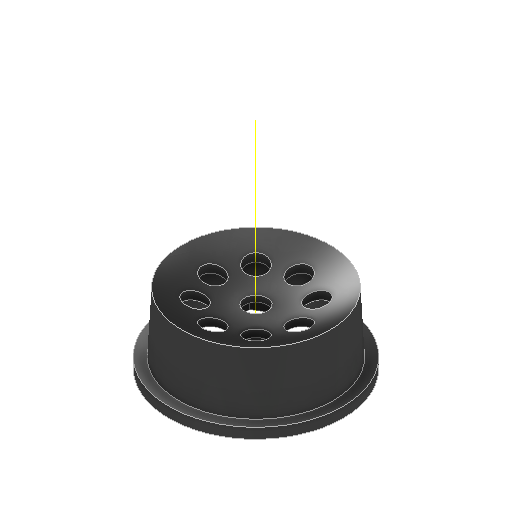
# Autodesk Inventor part: RIM ver 1
Saved by Autodesk Inventor 2023 (Build 270158000, 158)
## iProperties
Created: 2023-03-21
Part Number: RIM ver 1
Material: Generic
Document SubType Name: Modeling
Designer: Juyoung Han
Density: 1 g/cm^3
Appearance: Glossy - Black
Author: Juyoung Han
Autodesk Inventor part; units mm, degrees
ref_plane "YZ Plane" through (0, 0, 0) normal (1, 0, 0) x (0, 1, 0)
ref_plane "XZ Plane" through (0, 0, 0) normal (0, 1, 0) x (-1, 0, 0)
ref_plane "XY Plane" through (0, 0, 0) normal (0, 0, 1) x (1, 0, 0)
sketch "Sketch1" plane through (0, 0, 0) normal (0, 0, 1) x (1, 0, 0)
  line L0 (68.5, -28.5) -> (70.5, -28.5)
  line L1 (70.5, -28.5) -> (70.5, -20)
  line L2 (68.5, -28.5) -> (68.5, -22.5)
  line L3 (68.5, -22.5) -> (66.5, -22.5)
  line L4 (66.5, -22.5) -> (66.5, -24.5)
  line L5 (66.5, -24.5) -> (59.5, -24.5)
  line L6 (70.5, -20) -> (62.5, -20)
  line L7 (62.5, -20) -> (59.9389, 28.8689)
  line L8 (62.5, -20) -> (70.5, -20) construction
  line L9 (9.25, 16.5) -> (9.25, 11.5)
  line L10 (19, 11.5) -> (19, 3.5)
  line L11 (12, 3.5) -> (12, 11.5)
  arc A0 (9.25, 16.5) -> (59.9582, 28.5) centre (9.25, 129.6385) ccw
  line L12 (12, 11.5) -> (9.25, 11.5)
  line L13 (9.25, 11.5) -> (12, 11.5)
  line L14 (19, 3.5) -> (12, 3.5)
  line L15 (59.5, -24.5) -> (57.5607, 12.5037)
  line L16 (59.5, -24.5) -> (96.5545, -24.5) construction
  line L17 (57.5607, 12.5037) -> (57.1249, 20.8194)
  arc A1 (19, 11.5) -> (57.1249, 20.8194) centre (19, 94.1424) ccw
  line L18 (0, -60.1277) -> (0, 161.2662) projected
  point P0 (0, 0)
  point P1 (9.25, 14)
  dimension "d4" = 6
  dimension "d5" = 2
  dimension "d6" = 2
  dimension "d7" = 7
  dimension "d8" = 8
  dimension "d9" = 8.5
  dimension "d10" = 2
  dimension "d11" = 48.936
  dimension "d12" = 93
  dimension "d17" = 8
  dimension "d23" = 93
  constraints: 36 end point, 5 perpendicular, 4 horizontal, 4 point on circle, 2 centre point, 2 point on line, 1 equal length, 1 midpoint, 1 parallel, 1 vertical
  measures "d4" distance of L0.start L2.end
  measures "d5" distance of L2.end L3.end
  measures "d6" distance of L3.end L4.end
  measures "d7" distance of L4.end L5.end
  measures "d8" distance of L1.end L6.end
  measures "d9" distance between parallel lines of L0 L6
  measures "d10" distance between parallel lines of L1 L2
  measures "d11" distance of L6.end L7.end
  measures "d12" angle of L8 L7
  measures "d17" distance of L10.start L10.end
  measures "d23" angle of L16 L15
revolve "Revolution1" add sketch "Sketch1" angle 360 about axis through (0, -10, 0) along (0, 1, 0)
sketch "Sketch2" plane through (0, 3.5, 0) normal (0, -1, 0) x (1, 0, 0)
  circle A0 centre (0, 0) radius 12 projected
  circle A1 centre (0, 0) radius 19 projected
  line L0 (12, 6.9282) -> (12, -6.9282)
  line L1 (12, -6.9282) -> (0, -13.8564)
  line L2 (0, -13.8564) -> (-12, -6.9282)
  line L3 (-12, -6.9282) -> (-12, 6.9282)
  line L4 (-12, 6.9282) -> (0, 13.8564)
  line L5 (0, 13.8564) -> (12, 6.9282)
  point P0 (10.3923, -6)
  dimension "d47" = 24
  dimension "d48" = 0
  constraints: 12 end point, 2 coincident, 15 other
  measures "d47" distance between parallel lines of L4 L1
  measures "d48" horizontal distance of point (0, 0) L4.end
sketch "Sketch3" plane through (0, 3.5, 0) normal (0, -1, 0) x (1, 0, 0)
  circle A0 centre (0, 35) radius 8.75
  circle A1 centre (-24.7487, 24.7487) radius 8.75
  circle A2 centre (-35, 0) radius 8.75
  circle A3 centre (-24.7487, -24.7487) radius 8.75
  circle A4 centre (0, -35) radius 8.75
  circle A5 centre (24.7487, -24.7487) radius 8.75
  circle A6 centre (35, 0) radius 8.75
  circle A7 centre (24.7487, 24.7487) radius 8.75
  point P0 (0, 0)
  dimension "d26" = 17.5
  dimension "d27" = 35
  dimension "d30" = 360
  constraints: 8 centre point, 17 other
  measures "d26" diameter of A0
  measures "d27" distance of A0.centre point (0, 0)
extrude "Extrusion1" cut sketch "Sketch3" against normal through all
sketch "Sketch4" plane through (0, -24.5, 0) normal (0, -1, 0) x (1, 0, 0)
  circle A0 centre (-63, 0) radius 2.25
  circle A1 centre (-50.9681, -37.0305) radius 2.25
  circle A2 centre (-19.4681, -59.9166) radius 2.25
  circle A3 centre (19.4681, -59.9166) radius 2.25
  circle A4 centre (50.9681, -37.0305) radius 2.25
  circle A5 centre (63, 0) radius 2.25
  circle A6 centre (50.9681, 37.0305) radius 2.25
  circle A7 centre (19.4681, 59.9166) radius 2.25
  circle A8 centre (-19.4681, 59.9166) radius 2.25
  circle A9 centre (-50.9681, 37.0305) radius 2.25
  circle A10 centre (-63, 0) radius 1.25
  circle A11 centre (-50.9681, -37.0305) radius 1.25
  circle A12 centre (-19.4681, -59.9166) radius 1.25
  circle A13 centre (19.4681, -59.9166) radius 1.25
  circle A14 centre (50.9681, -37.0305) radius 1.25
  circle A15 centre (63, 0) radius 1.25
  circle A16 centre (50.9681, 37.0305) radius 1.25
  circle A17 centre (19.4681, 59.9166) radius 1.25
  circle A18 centre (-19.4681, 59.9166) radius 1.25
  circle A19 centre (-50.9681, 37.0305) radius 1.25
  point P0 (0, 0)
  dimension "d34" = 4.5
  dimension "d35" = 63
  dimension "d38" = 360
  dimension "d40" = 2.5
  dimension "d43" = 360
  constraints: 20 centre point, 1 coincident, 42 other
  measures "d34" diameter of A0
  measures "d35" distance of point (0, 0) A0.centre
  measures "d40" diameter of A10
extrude "Extrusion2" add sketch "Sketch4" along normal blind 2
extrude "Extrusion3" cut sketch "Sketch2" against normal blind 8 contours A0 | L0 L1 A0 | A0 L5 L0 | A0 L4 L5 | L1 L2 A0 | A0 L3 L4 | L2 L3 A0
body "Solid1"
